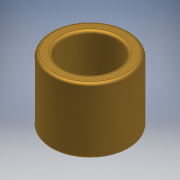
# Autodesk Inventor part: Bague
Saved by Autodesk Inventor 2017 (Build 210142000, 142)
## iProperties
Company: FABLAB FrenchMakers
Part Number: Bague
Material: Laiton, jaune doux
Document SubType Name: Modeling
Designer: FABLAB FrenchMakers
Density: 8.47 g/cm^3
Appearance: Laiton - Satiné
Mass: 5.26475 g
Surface Area: 7.27015 cm^2
Volume: 0.621577 cm^3
Stock Number: 1400-01-22
Project: 1400-PopCorn Machine
Author: Adrien MARY
Autodesk Inventor part; units mm, degrees
ref_plane "YZ Plane" through (0, 0, 0) normal (1, 0, 0) x (0, 1, 0)
ref_plane "XZ Plane" through (0, 0, 0) normal (0, 1, 0) x (-1, 0, 0)
ref_plane "XY Plane" through (0, 0, 0) normal (0, 0, 1) x (1, 0, 0)
sketch "Esquisse1" plane through (0, 0, 0) normal (0, 0, 1) x (1, 0, 0)
  circle A0 centre (0, 0) radius 4
  circle A1 centre (0, 0) radius 6
  dimension "d0" = 8
  dimension "d1" = 12
  constraints: 2 centre point, 2 coincident
  measures "d0" diameter of A0
  measures "d1" diameter of A1
extrude "Extrusion1" add sketch "Esquisse1" along normal mid plane 10
fillet "Congé1" radius 0.5 4 edges at (-4, 0, 5) (-6, 0, 5) (-6, 0, -5) (-4, 0, -5)
equation "\"nombredor\" = 1.61803"
equation "\"pi\" = 3.141593"
